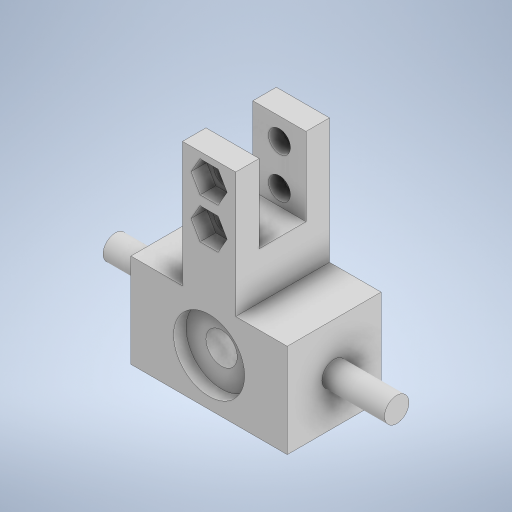
# Autodesk Inventor part: L0wer_battery
Saved by Autodesk Inventor 2024 (Build 280153000, 153)
## iProperties
Created: 2024-11-10
Part Number: L0wer_battery
Material: Generic
Document SubType Name: Modeling
Designer: manas
Density: 1 g/cm^3
Appearance: Default
Author: manas
Autodesk Inventor part; units mm, degrees
ref_plane "YZ Plane" through (0, 0, 0) normal (1, 0, 0) x (0, 1, 0)
ref_plane "XZ Plane" through (0, 0, 0) normal (0, 1, 0) x (-1, 0, 0)
ref_plane "XY Plane" through (0, 0, 0) normal (0, 0, 1) x (1, 0, 0)
sketch "Sketch1" plane through (0, 0, 0) normal (1, 0, 0) x (0, 1, 0)
  line L0 (-15, 15) -> (15, 15)
  line L1 (15, 15) -> (15, -15)
  line L2 (15, -15) -> (-15, -15)
  line L3 (-15, -15) -> (-15, 15)
  line L4 (-15, 15) -> (15, -15) construction
  line L5 (15, 15) -> (-15, -15) construction
  point P0 (0, 0)
  dimension "d0" = 30
  dimension "d1" = 30
  constraints: 12 end point, 2 midpoint, 2 parallel, 1 horizontal, 1 perpendicular
  measures "d0" distance of L1.end L2.end
  measures "d1" distance of L0.end L1.end
extrude "Extrusion1" add sketch "Sketch1" along normal blind 50
sketch "Sketch2" plane through (50, 0, 0) normal (1, 0, 0) x (0, 0, -1)
  circle A0 centre (0, 0) radius 3.9
  dimension "d5" = 7.8
  constraints: 1 centre point
  measures "d5" diameter of A0
extrude "Extrusion2" add sketch "Sketch2" along normal blind 20 and the other way blind 70
sketch "Sketch3" plane through (0, 15, 15) normal (0, 1, 0) x (1, 0, 0)
  line L0 (16.5, 30) -> (33.5, 30)
  line L1 (33.5, 30) -> (33.5, 0)
  line L2 (33.5, 0) -> (16.5, 0)
  line L3 (16.5, 0) -> (16.5, 30)
  line L4 (16.5, 30) -> (33.5, 0) construction
  line L5 (33.5, 30) -> (16.5, 0) construction
  point P0 (0, 15)
  point P1 (25, 15)
  dimension "d10" = 17
  dimension "d11" = 30
  constraints: 12 end point, 2 midpoint, 2 parallel, 1 horizontal, 1 perpendicular
  measures "d10" distance of L1.end L2.end
  measures "d11" distance of L0.end L1.end
extrude "Extrusion3" add sketch "Sketch3" along normal blind 40
sketch "Sketch4" plane through (0, -15, -15) normal (0, -1, 0) x (1, 0, 0)
  point P0 (0, 15)
sketch "Sketch5" plane through (0, -15, 15) normal (0, 0, 1) x (1, 0, 0)
  line L0 (0, 15) -> (50, 15)
  line L1 (50, 30) -> (50, 0) projected
  circle A0 centre (25, 15) radius 5
  dimension "d14" = 10
  constraints: 2 end point, 2 midpoint, 1 centre point
  measures "d14" diameter of A0
extrude "Extrusion4" cut sketch "Sketch5" against normal through all
sketch "Sketch6" plane through (0, -15, -15) normal (0, 0, -1) x (-1, 0, 0)
  point P0 (0, 15)
sketch "Sketch7" plane through (0, -15, 15) normal (0, 0, 1) x (1, 0, 0)
  circle A0 centre (25, 15) radius 5 projected
  circle A1 centre (25, 15) radius 11.35
  point P0 (0, 15)
  dimension "d17" = 22.7
  constraints: 1 centre point, 1 coincident
  measures "d17" diameter of A1
extrude "Extrusion5" cut sketch "Sketch7" against normal blind 4
sketch "Sketch8" plane through (0, 55, 15) normal (0, 1, 0) x (1, 0, 0)
  line L0 (16.5, 0) -> (16.5, 30) projected
  line L1 (16.5, 0) -> (33.5, 0) projected
  line L2 (16.5, 30) -> (33.5, 0)
  line L3 (33.5, 30) -> (33.5, 0) projected
  line L4 (16.5, 22.5) -> (33.5, 22.5)
  line L5 (33.5, 22.5) -> (33.5, 7.5)
  line L6 (33.5, 7.5) -> (16.5, 7.5)
  line L7 (16.5, 7.5) -> (16.5, 22.5)
  line L8 (16.5, 22.5) -> (33.5, 7.5) construction
  line L9 (33.5, 22.5) -> (16.5, 7.5) construction
  point P0 (0, 15)
  point P1 (25, 15)
  dimension "d20" = 15
  constraints: 14 end point, 3 midpoint, 2 parallel, 1 horizontal, 1 perpendicular, 1 point on line
  measures "d20" distance of L4.end L5.end
extrude "Extrusion6" cut sketch "Sketch8" against normal blind 25 contours L0 L4 L2 L6 | L2 L4 L3 L6
sketch "Sketch9" plane through (16.5, 55, -7.5) normal (0, 0, 1) x (1, 0, 0)
  line L0 (17, 0) -> (0, 0) projected
  line L1 (8.5, 0) -> (8.5, -25)
  line L2 (8.5, 0) -> (8.5, -7)
  line L3 (8.5, -7) -> (8.5, -25)
  line L4 (8.5, -25) -> (8.5, -20)
  circle A0 centre (8.5, -7) radius 3.5
  circle A1 centre (8.5, -20) radius 3.5
  point P0 (-16.5, -55)
  dimension "d23" = 25
  dimension "d24" = 7
  dimension "d25" = 5
  dimension "d26" = 7
  dimension "d27" = 7
  constraints: 8 end point, 2 centre point, 2 coincident, 2 point on line, 1 collinear, 1 midpoint, 1 vertical
  measures "d23" distance of L1.start L1.end
  measures "d24" distance of L1.start L2.end
  measures "d25" distance of L1.end L4.end
  measures "d26" diameter of A0
  measures "d27" diameter of A1
extrude "Extrusion7" cut sketch "Sketch9" along normal mid plane 100
sketch "Sketch10" plane through (0, -15, 15) normal (0, 0, 1) x (1, 0, 0)
  circle A0 centre (25, 63) radius 3.5 projected
  line L0 (30.7735, 63) -> (27.8868, 58)
  line L1 (27.8868, 58) -> (22.1132, 58)
  line L2 (22.1132, 58) -> (19.2265, 63)
  line L3 (19.2265, 63) -> (22.1132, 68)
  line L4 (22.1132, 68) -> (27.8868, 68)
  line L5 (27.8868, 68) -> (30.7735, 63)
  circle A1 centre (25, 50) radius 3.5 projected
  line L6 (30.7735, 50) -> (27.8868, 45)
  line L7 (27.8868, 45) -> (22.1132, 45)
  line L8 (22.1132, 45) -> (19.2265, 50)
  line L9 (19.2265, 50) -> (22.1132, 55)
  line L10 (22.1132, 55) -> (27.8868, 55)
  line L11 (27.8868, 55) -> (30.7735, 50)
  point P0 (0, 15)
  dimension "d30" = 10
  dimension "d31" = 10
  constraints: 24 end point, 2 coincident, 26 other
  measures "d30" distance between parallel lines of L1 L4
  measures "d31" distance between parallel lines of L7 L10
extrude "Extrusion8" cut sketch "Sketch10" against normal blind 5
sketch "Sketch11" plane through (0, -15, -15) normal (0, 0, -1) x (-1, 0, 0)
  circle A0 centre (-25, 63) radius 3.5 projected
  circle A1 centre (-25, 63) radius 5.25
  circle A2 centre (-25, 50) radius 3.5 projected
  circle A3 centre (-25, 50) radius 5.25
  point P0 (0, 15)
  dimension "d34" = 10.5
  dimension "d35" = 10.5
  constraints: 2 centre point, 2 coincident
  measures "d34" diameter of A1
  measures "d35" diameter of A3
extrude "Extrusion9" cut sketch "Sketch11" against normal blind 3 contours A0 | A1 | A2 | A3
body "Solid1"
